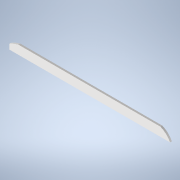
# Autodesk Inventor part: HolzLatteLinks
Saved by Autodesk Inventor 2020.3 (Build 243373010, 373A)
## iProperties
Created: 2021-02-05
Part Number: HolzLatteLinks
Material: Generisch
Document SubType Name: Modeling
Designer: Stefan
Density: 1 g/cm^3
Appearance: Vorgabe
Author: Stefan
Autodesk Inventor part; units mm, degrees
ref_plane "YZ Plane" through (0, 0, 0) normal (1, 0, 0) x (0, 1, 0)
ref_plane "XZ Plane" through (0, 0, 0) normal (0, 1, 0) x (-1, 0, 0)
ref_plane "XY Plane" through (0, 0, 0) normal (0, 0, 1) x (1, 0, 0)
sketch "Skizze1" plane through (0, 0, 0) normal (0, 0, 1) x (1, 0, 0)
  line L0 (-793.3777, 415) -> (953.6057, 415)
  arc A0 (953.6057, 415) -> (850.9934, 510) centre (775, 325) ccw
  line L1 (850.9934, 510) -> (-683.5127, 510)
  arc A1 (-683.5127, 510) -> (-793.3777, 460.1286) centre (-575, 125) ccw
  line L2 (-793.3777, 460.1286) -> (-793.3777, 415)
  line L3 (-793.3777, 460.1286) -> (-793.3777, 415)
  line L4 (-793.3777, 415) -> (953.6057, 415)
  arc A2 (953.6057, 415) -> (850.9934, 510) centre (775, 325) ccw
  line L5 (850.9934, 510) -> (-683.5127, 510)
  arc A3 (-683.5127, 510) -> (-793.3777, 460.1286) centre (-575, 125) ccw
  line L6 (-793.3777, 460.1286) -> (-793.3777, 415)
  arc A4 (953.6057, 415) -> (850.9934, 510) centre (775, 325) ccw
  line L7 (850.9934, 510) -> (-683.5127, 510)
  arc A5 (-683.5127, 510) -> (-793.3777, 460.1286) centre (-575, 125) ccw
  line L8 (953.6057, 415) -> (-793.3777, 415)
  point P0 (0, 0)
  point P1 (-793.3777, 460.1286)
  constraints: 18 end point, 12 point on circle, 6 centre point
extrude "Extrusion1" add sketch "Skizze1" along normal blind 20
sketch "Skizze2" plane through (-793.3777, 415, 0) normal (0, -1, 0) x (1, 0, 0)
  line L0 (-109.2775, 0) -> (-109.2775, 20)
  arc A0 (0, 0) -> (12.9517, 20) centre (-45.298, 43.5278) ccw
  line L1 (-109.2775, 0) -> (12.9517, 0)
  line L2 (0, -20) -> (-109.2775, -20)
  line L3 (-109.2775, 20) -> (12.9517, 20)
  line L4 (0, 0) -> (0, 20) projected
  point P0 (793.3777, 0)
  point P1 (-109.2775, 0)
  point P2 (0, 0)
  point P3 (12.9517, 20)
  dimension "d5" = 62.8218
  dimension "d6" = 90
  dimension "d7" = 20
  dimension "d8" = 20
  dimension "d9" = 0
  dimension "d11" = 122.2292
  dimension "d12" = 0
  dimension "d13" = 122.2292
  dimension "d14" = 122.2292
  dimension "d15" = 20
  dimension "d16" = 109.2776
  dimension "d17" = 109.2776
  dimension "d18" = 0
  dimension "d19" = 20
  dimension "d20" = 0
  dimension "d21" = 0
  constraints: 8 end point, 2 point on circle, 1 centre point, 1 horizontal, 1 parallel, 1 vertical
  measures "d5" radius of A0
  measures "d6" angle of L3 L0
  measures "d7" distance between parallel lines of L1 L2
  measures "d8" distance from line of point (793.378, 0) L3
  measures "d9" distance from line of point (793.378, 0) L1
  measures "d11" distance from line of L3.end L0
  measures "d12" distance from line of A0.end L3
  measures "d13" distance from line of A0.end L0
  measures "d14" distance from line of L1.end L0
  measures "d15" distance from line of A0.start L3
  measures "d16" distance from line of A0.start L0
  measures "d17" distance from line of L2.start L0
  measures "d18" distance from line of L1.start L0
  measures "d19" distance from line of L0.start L3
  measures "d20" distance from line of L2.end L0
  measures "d21" distance from line of L4 A0.start
extrude "Extrusion3" cut sketch "Skizze2" against normal through all
